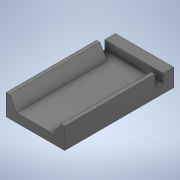
# Autodesk Inventor part: kicker_cover001
Saved by Autodesk Inventor 2020 (Build 240168000, 168)
## iProperties
Created: 2024-02-08
Part Number: kicker_cover001
Material: Типовые
Document SubType Name: Modeling
Designer: 4s
Density: 1 g/cm^3
Appearance: Гладкая — черная
Author: 4s
Autodesk Inventor part; units mm, degrees
ref_plane "YZ Plane" through (0, 0, 0) normal (1, 0, 0) x (0, 1, 0)
ref_plane "XZ Plane" through (0, 0, 0) normal (0, 1, 0) x (-1, 0, 0)
ref_plane "XY Plane" through (0, 0, 0) normal (0, 0, 1) x (1, 0, 0)
sketch "Эскиз1" plane through (0, 0, 0) normal (0, 1, 0) x (-1, 0, 0)
  line L0 (-8.25, 15.4) -> (8.25, 15.4)
  line L1 (8.25, 15.4) -> (8.25, -15.4)
  line L2 (8.25, -15.4) -> (-8.25, -15.4)
  line L3 (-8.25, -15.4) -> (-8.25, 15.4)
  line L4 (-8.25, 15.4) -> (8.25, -15.4) construction
  line L5 (8.25, 15.4) -> (-8.25, -15.4) construction
  point P0 (0, 0)
  dimension "d0" = 30.8
  dimension "d1" = 16.5
  constraints: 12 end point, 2 midpoint, 2 parallel, 1 horizontal, 1 perpendicular
  measures "d0" distance of L0.end L1.end
  measures "d1" distance of L1.end L2.end
extrude "Выдавливание1" add sketch "Эскиз1" along normal blind 2.5
sketch "Эскиз2" plane through (-8.25, 0, 15.4) normal (0, 0, 1) x (1, 0, 0)
  line L0 (0, 0) -> (16.5, 0) construction
  line L1 (16.5, 0) -> (16.5, 2.5) construction
  line L2 (0, 2.5) -> (16.5, 2.5) construction
  line L3 (0, 0) -> (0, 2.5) construction
  line L4 (0, 2.5) -> (0, 6)
  line L5 (0, 6) -> (1, 6)
  line L6 (0, 2.5) -> (3, 2.5)
  line L7 (0, 2.5) -> (16.5, 2.5) construction
  line L8 (3, 2.5) -> (1, 6)
  line L9 (8.25, 0) -> (8.25, 2.5) construction
  line L10 (16.5, 2.5) -> (16.5, 6)
  line L11 (16.5, 6) -> (15.5, 6)
  line L12 (16.5, 2.5) -> (13.5, 2.5)
  line L13 (13.5, 2.5) -> (15.5, 6)
  dimension "d4" = 3.5
  dimension "d5" = 1
  dimension "d6" = 3
  constraints: 18 end point, 3 symmetric about line, 1 midpoint, 1 perpendicular, 1 point on line, 1 vertical
  measures "d4" distance of L2.start L4.end
  measures "d5" distance of L4.end L5.end
  measures "d6" distance of L2.start L6.end
extrude "Выдавливание2" add sketch "Эскиз2" against normal blind 25.5
sketch "Эскиз3" plane through (8.25, 0, -15.4) normal (0, 0, -1) x (-1, 0, 0)
  line L0 (0, 0) -> (16.5, 0) construction
  line L1 (16.5, 0) -> (16.5, 2.5) construction
  line L2 (0, 2.5) -> (16.5, 2.5) projected
  line L3 (0, 0) -> (0, 2.5) construction
  line L4 (3, 2.5) -> (0, 2.5) projected
  line L5 (16.5, 0) -> (16.5, 6) construction
  line L6 (0, 2.5) -> (16.5, 2.5)
  line L7 (16.5, 2.5) -> (16.5, 5)
  line L8 (16.5, 5) -> (0, 5)
  line L9 (0, 5) -> (0, 2.5)
  point P0 (8.25, 0)
  dimension "d9" = 2.5
  constraints: 8 end point, 2 parallel, 1 horizontal, 1 perpendicular, 1 point on line
  measures "d9" distance of L7.end L6.end
extrude "Выдавливание3" add sketch "Эскиз3" against normal blind 3
